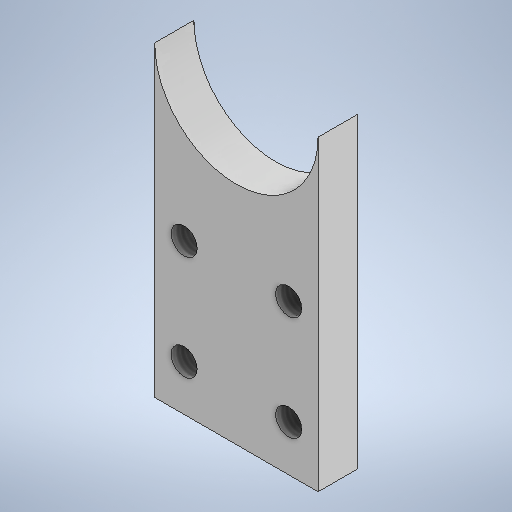
# Autodesk Inventor part: Clamp
Saved by Autodesk Inventor 2025.3 (Build 293356000, 356)
## iProperties
Created: 2026-04-19
Part Number: Clamp
Material: Generic
Document SubType Name: Modeling
Designer: logien
Density: 1 g/cm^3
Appearance: Default
Author: logien
Autodesk Inventor part; units mm, degrees
ref_plane "YZ Plane" through (0, 0, 0) normal (1, 0, 0) x (0, 1, 0)
ref_plane "XZ Plane" through (0, 0, 0) normal (0, 1, 0) x (-1, 0, 0)
ref_plane "XY Plane" through (0, 0, 0) normal (0, 0, 1) x (1, 0, 0)
sketch "Sketch1" plane through (0, 0, 0) normal (0, 0, 1) x (1, 0, 0)
  line L0 (0, 0) -> (25, 0)
  line L1 (0, 0) -> (0, -47)
  line L2 (0, -47) -> (25, -47)
  line L3 (25, -47) -> (25, 0)
  circle A0 centre (12.5, 0) radius 12.5
  dimension "d0" = 25
  dimension "d1" = 47
  constraints: 8 end point, 2 perpendicular, 1 centre point, 1 horizontal, 1 midpoint, 1 tangent, 1 vertical
  measures "d0" distance of L0.start L0.end
  measures "d1" distance of L0.start L1.end
extrude "Extrusion1" add sketch "Sketch1" along normal blind 6 contours A0 L3 L2 L1
sketch "Sketch2" plane through (0, 0, 6) normal (0, 0, 1) x (1, 0, 0)
  circle A0 centre (4.5, -24) radius 2
  circle A1 centre (20.5, -24) radius 2
  circle A2 centre (4.5, -40) radius 2
  circle A3 centre (20.5, -40) radius 2
  line L0 (0, -47) -> (25, -47) projected
  line L1 (0, 0) -> (0, -47) projected
  line L2 (25, -47) -> (25, 0) projected
  dimension "d16" = 4
  dimension "d17" = 4
  dimension "d18" = 4
  dimension "d19" = 4
  dimension "d20" = 7
  dimension "d21" = 7
  dimension "d22" = 16
  dimension "d23" = 16
  dimension "d25" = 4.5
  dimension "d26" = 4.5
  dimension "d27" = 4.5
  dimension "d28" = 4.5
  constraints: 4 centre point
  measures "d16" diameter of A0
  measures "d17" diameter of A1
  measures "d18" diameter of A2
  measures "d19" diameter of A3
  measures "d20" distance from line of L0 A3.centre
  measures "d21" distance from line of L0 A2.centre
  measures "d22" distance of A0.centre A2.centre
  measures "d23" distance of A1.centre A3.centre
  measures "d25" distance from line of L1 A0.centre
  measures "d26" distance from line of L2 A1.centre
  measures "d27" distance from line of L2 A3.centre
  measures "d28" distance from line of L1 A2.centre
extrude "Extrusion2" cut sketch "Sketch2" against normal through all
thread "Thread1" size "M4x0.7" class "6H" standard "ANSI Metric M Profile" length 36
thread "Thread2" size "M4x0.7" class "6H" standard "ANSI Metric M Profile" length 36
thread "Thread3" size "M4x0.7" class "6H" standard "ANSI Metric M Profile" length 36
thread "Thread4" size "M4x0.7" class "6H" standard "ANSI Metric M Profile" length 36
body "Solid1"
